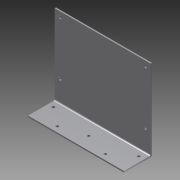
# Autodesk Inventor part: PowerDistributionStandmount
Saved by Autodesk Inventor 2012 (Build 160160000, 160)
## iProperties
Created: 2012-01-10
Part Number: PowerDistributionStandmount
Material: Default
Document SubType Name: Modeling
Designer: William
Density: 1 g/cm^3
Author: William
Autodesk Inventor part; units mm, degrees
ref_plane "YZ Plane" through (0, 0, 0) normal (1, 0, 0) x (0, 1, 0)
ref_plane "XZ Plane" through (0, 0, 0) normal (0, 1, 0) x (-1, 0, 0)
ref_plane "XY Plane" through (0, 0, 0) normal (0, 0, 1) x (1, 0, 0)
sketch "Sketch1" plane through (0, 0, 0) normal (0, 0, 1) x (1, 0, 0)
  line L0 (39.835, -215.3282) -> (-188.765, -215.3282)
  line L1 (-188.765, -215.3282) -> (-188.765, -22.2882)
  line L2 (-188.765, -22.2882) -> (39.835, -22.2882)
  line L3 (39.835, -22.2882) -> (39.835, -215.3282)
  point P0 (0, 0)
  dimension "d0" = 228.6
  dimension "d1" = 193.04
  constraints: 8 end point, 2 parallel, 1 horizontal, 1 perpendicular
  measures "d0" distance of L1.end L2.end
  measures "d1" distance of L0.end L1.end
extrude "Extrusion1" add sketch "Sketch1" along normal blind 3.175
sketch "Sketch2" plane through (0, 0, 3.175) normal (0, 0, 1) x (1, 0, 0)
  line L0 (-188.765, -215.3282) -> (39.835, -215.3282)
  line L1 (39.835, -215.3282) -> (39.835, -212.1532)
  line L2 (39.835, -212.1532) -> (-188.765, -212.1532)
  line L3 (-188.765, -212.1532) -> (-188.765, -215.3282)
  point P0 (0, 0)
  dimension "d4" = 228.6
  dimension "d5" = 3.175
  constraints: 8 end point, 2 parallel, 1 horizontal, 1 perpendicular
  measures "d4" distance of L2.end L1.end
  measures "d5" distance of L1.end L0.end
extrude "Extrusion2" add sketch "Sketch2" along normal blind 63.5
fillet "Fillet1" radius 3.175 2 edges at (-74.465, -212.1532, 3.175) (-74.465, -215.3282, 0)
sketch "Sketch3" plane through (-188.765, -212.1532, 66.675) normal (0, 1, 0) x (1, 0, 0)
  line L0 (0, 60.325) -> (228.6, 60.325) projected
  line L1 (0, 60.325) -> (0, 0) projected
  line L2 (0, 0) -> (228.6, 0) projected
  line L3 (228.6, 60.325) -> (228.6, 0) projected
  circle A0 centre (12.7, 47.625) radius 3.175
  circle A1 centre (114.3, 30.1625) radius 3.175
  circle A2 centre (215.9, 47.625) radius 3.175
  circle A3 centre (57.15, 12.7) radius 3.175
  circle A4 centre (171.45, 12.7) radius 3.175
  point P0 (188.765, 66.675)
  dimension "d9" = 6.35
  dimension "d10" = 6.35
  dimension "d11" = 6.35
  dimension "d12" = 6.35
  dimension "d13" = 6.35
  dimension "d14" = 12.7
  dimension "d15" = 12.7
  dimension "d16" = 12.7
  dimension "d17" = 12.7
  dimension "d18" = 114.3
  dimension "d19" = 228.6
  dimension "d20" = 57.15
  dimension "d21" = 12.7
  dimension "d22" = 12.7
  dimension "d23" = 57.15
  dimension "d24" = 30.1625
  dimension "d25" = 60.325
  constraints: 5 centre point
  measures "d9" diameter of A0
  measures "d10" diameter of A1
  measures "d11" diameter of A2
  measures "d12" diameter of A3
  measures "d13" diameter of A4
  measures "d14" distance from line of A0.centre L0
  measures "d15" distance from line of L1 A0.centre
  measures "d16" distance from line of L0 A2.centre
  measures "d17" distance from line of L3 A2.centre
  measures "d18" distance from line of L1 A1.centre
  measures "d19" distance of L1.end L2.end
  measures "d20" distance from line of L3 A4.centre
  measures "d21" distance from line of L2 A4.centre
  measures "d22" distance from line of L2 A3.centre
  measures "d23" distance from line of L1 A3.centre
  measures "d24" distance from line of L2 A1.centre
  measures "d25" distance of L0.end L2.end
extrude "Extrusion3" cut sketch "Sketch3" against normal blind 63.5 contours A0 | A1 | A2 | A3 | A4
sketch "Sketch4" plane through (0, 0, 3.175) normal (0, 0, 1) x (1, 0, 0)
  line L0 (39.835, -22.2882) -> (39.835, -208.9782) projected
  line L1 (-188.765, -22.2882) -> (39.835, -22.2882) projected
  line L2 (-188.765, -208.9782) -> (-188.765, -22.2882) projected
  circle A0 centre (-176.065, -34.9882) radius 3.175
  circle A1 centre (27.135, -34.9882) radius 3.175
  circle A2 centre (-176.065, -161.9882) radius 3.175
  circle A3 centre (27.135, -161.9882) radius 3.175
  point P0 (0, 0)
  dimension "d28" = 6.35
  dimension "d29" = 6.35
  dimension "d30" = 12.7
  dimension "d31" = 12.7
  dimension "d32" = 12.7
  dimension "d33" = 12.7
  dimension "d34" = 6.35
  dimension "d35" = 6.35
  dimension "d36" = 12.7
  dimension "d37" = 12.7
  dimension "d38" = 127
  dimension "d39" = 127
  constraints: 4 centre point
  measures "d28" diameter of A0
  measures "d29" diameter of A1
  measures "d30" distance from line of L1 A0.centre
  measures "d31" distance from line of L2 A0.centre
  measures "d32" distance from line of L1 A1.centre
  measures "d33" distance from line of L0 A1.centre
  measures "d34" diameter of A2
  measures "d35" diameter of A3
  measures "d36" distance from line of L2 A2.centre
  measures "d37" distance from line of L0 A3.centre
  measures "d38" distance of A2.centre A0.centre
  measures "d39" distance of A3.centre A1.centre
extrude "Extrusion4" cut sketch "Sketch4" against normal blind 63.5
equation "\"d18\" = 0.5 * d19"
equation "\"d20\" = 0.25 * d19"
equation "\"d22\" = d21"
equation "\"d23\" = d20"
equation "\"d24\" = 0.5 * d25"
equation "\"d37\" = d36"
equation "\"d39\" = d38"
body "Solid1"
